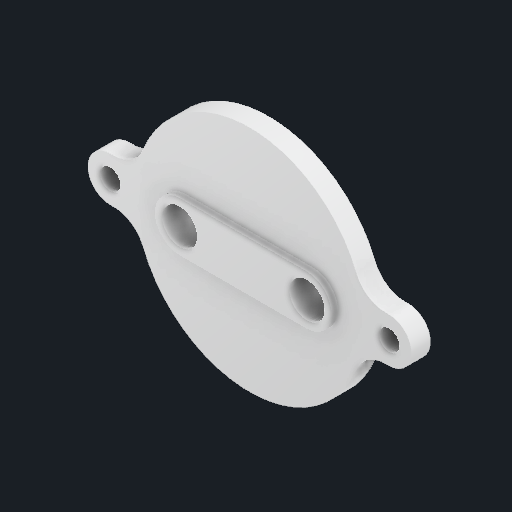
# Autodesk Inventor part: nema 14 cooler lid
Saved by Autodesk Inventor 2024.3 (Build 283343000, 343)
## iProperties
Created: 2024-10-05
Part Number: nema 14 cooler lid
Material: Aluminum 6061
Document SubType Name: Modeling
Designer: MFil
Mass: 2.98794 g
Surface Area: 23.8933 cm^2
Volume: 1.10664 cm^3
Density: 2.7 g/cm^3
Appearance: Aluminum - Flat
Author: MFil
Autodesk Inventor part; units mm, degrees
ref_plane "YZ Plane" through (0, 0, 0) normal (1, 0, 0) x (0, 1, 0)
ref_plane "XZ Plane" through (0, 0, 0) normal (0, 1, 0) x (-1, 0, 0)
ref_plane "XY Plane" through (0, 0, 0) normal (0, 0, 1) x (1, 0, 0)
sketch "Sketch1" plane through (0, 0, 0) normal (0, 0, 1) x (1, 0, 0)
  arc A0 (-13.0211, -6.6387) -> (-17.9871, -3.4929) centre (-17.6686, -8.4827) ccw projected
  arc A1 (-13.0211, -6.6387) -> (20.4411, -6.6387) centre (3.71, 0) ccw projected
  arc A2 (25.4071, -3.4929) -> (20.4411, -6.6387) centre (25.0886, -8.4827) ccw projected
  arc A3 (25.4071, -3.4929) -> (25.4071, 3.4929) centre (25.63, 0) ccw projected
  arc A4 (20.4411, 6.6387) -> (25.4071, 3.4929) centre (25.0886, 8.4827) ccw projected
  arc A5 (20.4411, 6.6387) -> (-13.0211, 6.6387) centre (3.71, 0) ccw projected
  arc A6 (-17.9871, 3.4929) -> (-13.0211, 6.6387) centre (-17.6686, 8.4827) ccw projected
  arc A7 (-17.9871, 3.4929) -> (-17.9871, -3.4929) centre (-18.21, 0) ccw projected
  circle A8 centre (3.71, 0) radius 17.1 projected
  circle A9 centre (-18.21, 0) radius 1.25 projected
  circle A10 centre (25.63, 0) radius 1.25 projected
  arc A11 (-9.29, 0) -> (-3.29, 0) centre (-6.29, 0) ccw projected
  arc A12 (1.3159, 6.5778) -> (-3.29, 0) centre (3.71, 0) ccw projected
  arc A13 (2.5208, 2.7543) -> (1.3159, 6.5778) centre (2.0021, 4.6924) ccw projected
  arc A14 (2.5208, 2.7543) -> (5.9674, -12.8025) centre (4.5827, -4.9491) ccw projected
  arc A15 (5.9674, -12.8025) -> (16.71, 0) centre (3.71, 0) ccw projected
  arc A16 (16.71, 0) -> (10.71, 0) centre (13.71, 0) ccw projected
  arc A17 (6.1041, -6.5778) -> (10.71, 0) centre (3.71, 0) ccw projected
  arc A18 (4.8992, -2.7543) -> (6.1041, -6.5778) centre (5.4179, -4.6924) ccw projected
  arc A19 (4.8992, -2.7543) -> (1.4526, 12.8025) centre (2.8373, 4.9491) ccw projected
  arc A20 (1.4526, 12.8025) -> (-9.29, 0) centre (3.71, 0) ccw projected
  circle A21 centre (13.71, 0) radius 2.75
  circle A22 centre (-6.29, 0) radius 2.75
  circle A23 centre (-18.21, 0) radius 1.6
  circle A24 centre (25.63, 0) radius 1.6
  point P0 (0, 0)
  dimension "d0" = 5.5
  dimension "d1" = 5.5
  dimension "d21" = 3.2
  dimension "d22" = 3.2
  constraints: 4 centre point, 4 coincident
  measures "d0" diameter of A21
  measures "d1" diameter of A22
  measures "d21" diameter of A23
  measures "d22" diameter of A24
extrude "Extrusion1" add sketch "Sketch1" along normal blind 1 contours A0 A7 A6 A5 A4 A3 A2 A1 | A8 | A20 A19 A18 A17 A16 A15 A14 A13 A12 A11
sketch "Sketch2" plane through (0, 0, 1) normal (0, 0, 1) x (1, 0, 0)
  arc A0 (20.4411, 6.6387) -> (25.4071, 3.4929) centre (25.0886, 8.4827) ccw projected
  arc A1 (20.4411, 6.6387) -> (-13.0211, 6.6387) centre (3.71, 0) ccw projected
  arc A2 (-17.9871, 3.4929) -> (-13.0211, 6.6387) centre (-17.6686, 8.4827) ccw projected
  arc A3 (-17.9871, 3.4929) -> (-17.9871, -3.4929) centre (-18.21, 0) ccw projected
  arc A4 (-13.0211, -6.6387) -> (-17.9871, -3.4929) centre (-17.6686, -8.4827) ccw projected
  arc A5 (-13.0211, -6.6387) -> (20.4411, -6.6387) centre (3.71, 0) ccw projected
  arc A6 (25.4071, -3.4929) -> (20.4411, -6.6387) centre (25.0886, -8.4827) ccw projected
  arc A7 (25.4071, -3.4929) -> (25.4071, 3.4929) centre (25.63, 0) ccw projected
  circle A8 centre (-6.29, 0) radius 2.75 projected
  circle A9 centre (13.71, 0) radius 2.75 projected
  line L0 (29.13, 0) -> (-21.71, 0) construction
  line L1 (25.63, 3.5) -> (-18.21, 3.5)
  line L2 (-18.21, -3.5) -> (25.63, -3.5)
  arc A10 (25.63, -3.5) -> (25.63, 3.5) centre (25.63, 0) ccw
  arc A11 (-18.21, 3.5) -> (-18.21, -3.5) centre (-18.21, 0) ccw
  arc A12 (-11.162, -5.901) -> (18.582, -5.901) centre (3.71, 0) ccw
  arc A13 (-11.162, -5.901) -> (-18.1145, -1.497) centre (-17.6686, -8.4827) ccw
  arc A14 (-18.1145, 1.497) -> (-18.1145, -1.497) centre (-18.21, 0) ccw
  arc A15 (-18.1145, 1.497) -> (-11.162, 5.901) centre (-17.6686, 8.4827) ccw
  arc A16 (18.582, 5.901) -> (-11.162, 5.901) centre (3.71, 0) ccw
  arc A17 (18.582, 5.901) -> (25.5345, 1.497) centre (25.0886, 8.4827) ccw
  arc A18 (25.5345, -1.497) -> (25.5345, 1.497) centre (25.63, 0) ccw
  arc A19 (25.5345, -1.497) -> (18.582, -5.901) centre (25.0886, -8.4827) ccw
  circle A20 centre (16.5844, -5.5) radius 2
  circle A21 centre (-9.1772, -5.5) radius 2
  circle A22 centre (16.5972, 5.5) radius 2
  circle A23 centre (-9.1644, 5.5) radius 2
  circle A24 centre (-18.21, 0) radius 1.6 projected
  circle A25 centre (25.63, 0) radius 1.6 projected
  point P0 (0, 0)
  point P1 (3.71, 0)
  point P2 (-9.1772, -3.5)
  point P3 (16.5844, -3.5)
  point P4 (18.4236, -6.2857)
  point P5 (-10.9134, -6.4928)
  point P6 (16.5972, 3.5)
  point P7 (-9.1644, 3.5)
  point P8 (-11.0036, 6.2857)
  point P9 (18.3334, 6.4928)
  dimension "d4" = 7
  dimension "d5" = 2
  dimension "d6" = 4
  dimension "d7" = 4
  dimension "d8" = 4
  dimension "d9" = 4
  constraints: 24 point on circle, 14 centre point, 12 tangent, 8 end point, 2 point on line, 1 midpoint, 1 parallel, 7 other
  measures "d4" diameter of A11
  measures "d5" radial gap between concentric circles of A5 A12
  measures "d6" diameter of A20
  measures "d7" diameter of A21
  measures "d8" diameter of A22
  measures "d9" diameter of A23
extrude "Extrusion2" add sketch "Sketch2" along normal blind 2 contours A0 L1 A17 A16 A22 A15 A2 A1 | A0 A7 A6 L2 A19 A25 A17 L1 | A17 A25 A19 L2 A13 A24 A15 L1 | L1 A22 A16 A17 | L1 A15 A24 A13 L2 A4 A3 A2 | A15 A16 A23 L1 | A6 A5 A4 L2 A13 A12 A21 A19 | A19 A12 A20 L2 | L2 A21 A12 A13
sketch "Sketch3" plane through (0, 0, 3) normal (0, 0, 1) x (1, 0, 0)
  arc A0 (-17.9871, 3.4929) -> (-17.9871, -3.4929) centre (-18.21, 0) ccw projected
  arc A1 (-13.0211, -6.6387) -> (-17.9871, -3.4929) centre (-17.6686, -8.4827) ccw projected
  arc A2 (-13.0211, -6.6387) -> (20.4411, -6.6387) centre (3.71, 0) ccw projected
  arc A3 (25.4071, -3.4929) -> (20.4411, -6.6387) centre (25.0886, -8.4827) ccw projected
  arc A4 (25.4071, -3.4929) -> (25.4071, 3.4929) centre (25.63, 0) ccw projected
  arc A5 (20.4411, 6.6387) -> (25.4071, 3.4929) centre (25.0886, 8.4827) ccw projected
  arc A6 (20.4411, 6.6387) -> (-13.0211, 6.6387) centre (3.71, 0) ccw projected
  arc A7 (-17.9871, 3.4929) -> (-13.0211, 6.6387) centre (-17.6686, 8.4827) ccw projected
  line L0 (-9.1772, -3.5) -> (16.5844, -3.5) projected
  arc A8 (18.4236, -6.2857) -> (16.5844, -3.5) centre (16.5844, -5.5) ccw projected
  arc A9 (-10.9134, -6.4928) -> (18.4236, -6.2857) centre (3.71, 0) ccw projected
  arc A10 (-9.1772, -3.5) -> (-10.9134, -6.4928) centre (-9.1772, -5.5) ccw projected
  circle A11 centre (13.71, 0) radius 2.75 projected
  circle A12 centre (-6.29, 0) radius 2.75 projected
  arc A13 (16.5972, 3.5) -> (18.3334, 6.4928) centre (16.5972, 5.5) ccw projected
  line L1 (16.5972, 3.5) -> (-9.1644, 3.5) projected
  arc A14 (-11.0036, 6.2857) -> (-9.1644, 3.5) centre (-9.1644, 5.5) ccw projected
  arc A15 (18.3334, 6.4928) -> (-11.0036, 6.2857) centre (3.71, 0) ccw projected
  circle A16 centre (13.71, 0) radius 3.9
  circle A17 centre (-6.29, 0) radius 3.9
  line L2 (3.8229, -15.9996) -> (3.5971, 15.9996)
  line L3 (4.8229, -15.9925) -> (4.597, 16.0067)
  line L4 (2.823, -16.0067) -> (2.5971, 15.9925)
  point P0 (0, 0)
  point P1 (11.9895, 3.5)
  point P2 (15.4305, 3.5)
  point P3 (15.4305, -3.5)
  point P4 (11.9895, -3.5)
  point P5 (-4.5695, -3.5)
  point P6 (-8.0105, -3.5)
  point P7 (-8.0105, 3.5)
  point P8 (-4.5695, 3.5)
  point P9 (2.7347, -3.5)
  point P10 (2.8227, -15.9754)
  point P11 (4.8227, -15.9613)
  point P12 (4.7347, -3.5)
  point P13 (4.6853, 3.5)
  point P14 (4.5973, 15.9754)
  point P15 (2.5973, 15.9613)
  point P16 (2.6853, 3.5)
  dimension "d12" = 7.8
  dimension "d13" = 7.8
  dimension "d14" = 1
  dimension "d15" = 1
  constraints: 6 end point, 2 centre point, 2 coincident, 2 parallel, 2 point on circle
  measures "d12" diameter of A16
  measures "d13" diameter of A17
  measures "d14" distance between parallel lines of L2 L3
  measures "d15" distance between parallel lines of L2 L4
extrude "Extrusion3" add sketch "Sketch3" against normal up to surface (2 mm away) contours L0 A17 | A17 L1 | L4 L0 L2 A9 | L2 L0 L3 A9 | L4 A15 L2 L1 | L2 A15 L3 L1 | L0 A16 | A16 L1
extrude "Extrusion4" add sketch "Sketch3" along normal blind 1 contours A17 L1 L0 | L0 A17 | A17 L1 | A16 L1 L0 | L0 A16 | A16 L1
fillet "Fillet1" radius 2 16 edges at (15.4305, 3.5, 2) (11.9895, 3.5, 2) (-4.5695, 3.5, 2) (-8.0105, 3.5, 2) (15.4305, -3.5, 2) (11.9895, -3.5, 2) (-4.5695, -3.5, 2) (-8.0105, -3.5, 2) (2.7347, -3.5, 2) (4.7347, -3.5, 2) (2.6853, 3.5, 2) (4.6853, 3.5, 2) (2.5973, 15.9613, 2) (4.5973, 15.9754, 2) (2.8227, -15.9754, 2) (4.8227, -15.9613, 2)
move faces "Move2" translate (0, 0, 2) faces at (10.0093, 7.1393, 1) (-1.6209, 7.7859, 1) (-2.5893, -7.1393, 1) (9.0409, -7.7859, 1)
move faces "Move3" translate (0, 0, 1) faces at (3.71, 7.2157, 0)
move faces "Move4" translate (0, 0, 1) faces at (17.1889, 0.3111, 4) (-2.8377, 0.5305, 4)
move faces "Move5" translate (0, 0, 1) faces at (3.71, 7.7241, 3)
sketch "Sketch4" plane through (-6.29, 0, 5) normal (0, 0, 1) x (1, 0, 0)
  circle A0 centre (0, 0) radius 3.9 projected
  circle A1 centre (0, 0) radius 2.75 projected
  circle A2 centre (20, 0) radius 3.9 projected
  circle A3 centre (20, 0) radius 2.75 projected
  circle A4 centre (0, 0) radius 3.9 projected
  line L0 (0, 3.9) -> (20, 3.9)
  line L1 (20, 3.9) -> (20, -3.9)
  line L2 (20, -3.9) -> (0, -3.9)
  line L3 (0, -3.9) -> (0, 3.9)
  point P0 (6.29, 0)
  constraints: 8 end point, 2 parallel, 1 horizontal, 1 perpendicular, 1 vertical alignment, 3 other
extrude "Extrusion5" add sketch "Sketch4" against normal up to surface (1 mm away) contours A0 L0 A2 L2
equation "\"d12\" = d13"
body "Solid1"
